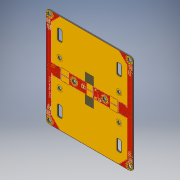
# Autodesk Inventor part: SolarPanel_PCB
Saved by Autodesk Inventor 2018 (Build 220112000, 112)
## iProperties
Created: 2018-11-29
Part Number: SolarPanel_PCB
Material: Epoxy Resin
Document SubType Name: Modeling
Designer: Bradley
Density: 1.14 g/cm^3
Appearance: Smooth - Dark Gray
Author: Bradley
Autodesk Inventor part; units mm, degrees
ref_plane "YZ Plane" through (0, 0, 0) normal (1, 0, 0) x (0, 1, 0)
ref_plane "XZ Plane" through (0, 0, 0) normal (0, 1, 0) x (-1, 0, 0)
ref_plane "XY Plane" through (0, 0, 0) normal (0, 0, 1) x (1, 0, 0)
sketch "Sketch1" plane through (0, 0, 0) normal (0, 1, 0) x (-1, 0, 0)
  line L0 (36.5, -45) -> (-36.5, -45)
  line L1 (-39.5, -42) -> (-39.5, 42)
  line L2 (-36.5, 45) -> (36.5, 45)
  line L3 (39.5, 42) -> (39.5, -42)
  line L4 (39.5, -45) -> (-39.5, 45) construction
  line L5 (-39.5, -45) -> (39.5, 45) construction
  arc A0 (39.5, 42) -> (36.5, 45) centre (36.5, 42) ccw
  arc A1 (36.5, -45) -> (39.5, -42) centre (36.5, -42) ccw
  arc A2 (-39.5, -42) -> (-36.5, -45) centre (-36.5, -42) ccw
  arc A3 (-36.5, 45) -> (-39.5, 42) centre (-36.5, 42) ccw
  circle A4 centre (36.5, 42) radius 1.65
  circle A5 centre (-36.5, 42) radius 1.65
  circle A6 centre (-36.5, -42) radius 1.65
  circle A7 centre (36.5, -42) radius 1.65
  line L6 (14, 0) -> (-14, 0) construction
  circle A8 centre (14, 0) radius 1.65
  circle A9 centre (-14, 0) radius 1.65
  line L7 (28, 35) -> (26, 35)
  line L8 (25, 34) -> (25, 26)
  line L9 (26, 25) -> (28, 25)
  line L10 (29, 26) -> (29, 34)
  line L11 (-26, 35) -> (-28, 35)
  line L12 (-29, 34) -> (-29, 26)
  line L13 (-28, 25) -> (-26, 25)
  line L14 (-25, 26) -> (-25, 34)
  line L15 (28, -25) -> (26, -25)
  line L16 (25, -26) -> (25, -34)
  line L17 (26, -35) -> (28, -35)
  line L18 (29, -34) -> (29, -26)
  line L19 (-26, -25) -> (-28, -25)
  line L20 (-29, -26) -> (-29, -34)
  line L21 (-28, -35) -> (-26, -35)
  line L22 (-25, -34) -> (-25, -26)
  line L23 (0, 45) -> (0, -45) construction
  arc A10 (29, 34) -> (28, 35) centre (28, 34) ccw
  arc A11 (26, 35) -> (25, 34) centre (26, 34) ccw
  arc A12 (25, 26) -> (26, 25) centre (26, 26) ccw
  arc A13 (28, 25) -> (29, 26) centre (28, 26) ccw
  arc A14 (26, -25) -> (25, -26) centre (26, -26) ccw
  arc A15 (29, -26) -> (28, -25) centre (28, -26) ccw
  arc A16 (28, -35) -> (29, -34) centre (28, -34) ccw
  arc A17 (25, -34) -> (26, -35) centre (26, -34) ccw
  arc A18 (-26, -35) -> (-25, -34) centre (-26, -34) ccw
  arc A19 (-26, 25) -> (-25, 26) centre (-26, 26) ccw
  arc A20 (-25, 34) -> (-26, 35) centre (-26, 34) ccw
  arc A21 (-28, 35) -> (-29, 34) centre (-28, 34) ccw
  arc A22 (-29, 26) -> (-28, 25) centre (-28, 26) ccw
  arc A23 (-28, -25) -> (-29, -26) centre (-28, -26) ccw
  arc A24 (-25, -26) -> (-26, -25) centre (-26, -26) ccw
  arc A25 (-29, -34) -> (-28, -35) centre (-28, -34) ccw
  point P0 (0, 0)
  point P1 (0, 0)
  point P2 (-25, 35)
  point P3 (-29, 25)
  point P4 (29, -25)
  point P5 (25, -35)
  point P6 (-25, -25)
  point P7 (-29, -35)
  dimension "d0" = 79
  dimension "d1" = 90
  dimension "d2" = 3
  dimension "d3" = 3.3
  dimension "d4" = 28
  dimension "d92" = 29
  dimension "d93" = 35
  dimension "d94" = 25
  dimension "d95" = 25
  dimension "d96" = 1
  constraints: 48 end point, 40 point on circle, 40 tangent, 28 point on line, 26 centre point, 23 equal radius, 10 parallel, 6 coincident, 6 horizontal, 6 midpoint, 5 perpendicular, 1 collinear, 3 other
  measures "d0" distance of L4.end L5.end
  measures "d1" distance of L5.end L4.start
  measures "d2" radius of A0
  measures "d3" diameter of A4
  measures "d4" distance of L6.start L6.end
  measures "d92" distance from line of L10 point (0, 0)
  measures "d93" distance from line of point (0, 0) L7
  measures "d94" distance from line of L9 point (0, 0)
  measures "d95" distance from line of point (0, 0) L8
  measures "d96" radius of A10
extrude "Extrusion1" add sketch "Sketch1" along normal mid plane 1
sketch "Sketch8" plane through (0, -0.5, 0) normal (0, -1, 0) x (1, 0, 0)
  line L0 (-39.5061, 45) -> (39.5061, 45) construction
  line L1 (39.5061, 45) -> (39.5061, -45) construction
  line L2 (39.5061, -45) -> (-39.5061, -45) construction
  line L3 (-39.5061, -45) -> (-39.5061, 45) construction
  line L4 (36.5, 45) -> (-36.5, 45) projected
  line L5 (-36.5, -45) -> (36.5, -45) projected
  point P0 (0, 0)
  point P1 (0, 45)
  constraints: 2 collinear, 2 midpoint, 2 other
decal "Decal3"
sketch "Sketch9" plane through (0, 0.5, 0) normal (0, 1, 0) x (1, 0, 0)
  line L0 (-36.5, -45) -> (36.5, -45) projected
  line L1 (36.5, 45) -> (-36.5, 45) projected
  line L2 (39.5061, -45) -> (-39.5061, -45) construction
  line L3 (-39.5061, -45) -> (-39.5061, 45) construction
  line L4 (-39.5061, 45) -> (39.5061, 45) construction
  line L5 (39.5061, 45) -> (39.5061, -45) construction
  point P0 (0, 0)
  point P1 (0, -45)
  point P2 (0, -45)
  constraints: 3 midpoint, 2 collinear, 2 other
decal "Decal4"
sketch "Sketch10" plane through (0, -0.5, 0) normal (0, -1, 0) x (1, 0, 0)
  point P0 (0, 0)
  point P1 (27, -12)
  point P2 (-27, -12)
  point P3 (-27, 12)
  point P4 (27, 12)
  constraints: 5 other
hole "Hole5" at (27, -0.5, -12) at (-27, -0.5, -12) at (-27, -0.5, 12) at (27, -0.5, 12) direction (0, 1, 0) diameter 3 end through all
sketch "Sketch11" plane through (0, -0.5, 0) normal (0, -1, 0) x (1, 0, 0)
  point P0 (0, 0)
  point P1 (-35.789, -39.813)
  point P2 (-37.211, -39.813)
  point P3 (-38.361, -40.648)
  point P4 (-38.8, -42)
  point P5 (-38.361, -43.352)
  point P6 (-37.211, -44.187)
  point P7 (-35.789, -44.187)
  point P8 (-34.639, -40.648)
  point P9 (-34.2, 42)
  point P10 (-34.639, 43.352)
  point P11 (-35.789, 44.187)
  point P12 (-37.211, 44.187)
  point P13 (-38.361, 43.352)
  point P14 (-38.8, 42)
  point P15 (-38.361, 40.648)
  point P16 (-37.211, 39.813)
  point P17 (-35.789, 39.813)
  point P18 (-34.639, 40.648)
  point P19 (38.8, 42)
  point P20 (38.361, 43.352)
  point P21 (37.211, 44.187)
  point P22 (35.789, 44.187)
  point P23 (34.639, 43.352)
  point P24 (34.2, 42)
  point P25 (34.639, 40.648)
  point P26 (35.789, 39.813)
  point P27 (37.211, 39.813)
  point P28 (38.361, 40.648)
  point P29 (-34.639, -43.352)
  point P30 (38.8, -42)
  point P31 (38.361, -40.648)
  point P32 (37.211, -39.813)
  point P33 (35.789, -39.813)
  point P34 (34.639, -40.648)
  point P35 (34.2, -42)
  point P36 (34.639, -43.352)
  point P37 (35.789, -44.187)
  point P38 (37.211, -44.187)
  point P39 (38.361, -43.352)
  point P40 (-34.2, -42)
  point P41 (-11.7, 0)
  point P42 (-12.139, 1.352)
  point P43 (-14.711, 2.187)
  point P44 (-15.861, 1.352)
  point P45 (-16.3, 0)
  point P46 (-15.861, -1.352)
  point P47 (-14.711, -2.187)
  point P48 (-13.289, -2.187)
  point P49 (-12.139, -1.352)
  point P50 (-13.289, 2.187)
  point P51 (16.3, 0)
  point P52 (15.861, 1.352)
  point P53 (14.711, 2.187)
  point P54 (13.289, 2.187)
  point P55 (12.139, 1.352)
  point P56 (11.7, 0)
  point P57 (12.139, -1.352)
  point P58 (13.289, -2.187)
  point P59 (14.711, -2.187)
  point P60 (15.861, -1.352)
  constraints: 61 other
hole "Hole6" at (-35.789, -0.5, -39.813) at (-37.211, -0.5, -39.813) at (-38.361, -0.5, -40.648) at (-38.8, -0.5, -42) at (-38.361, -0.5, -43.352) at (-37.211, -0.5, -44.187) at (-35.789, -0.5, -44.187) at (-34.639, -0.5, -40.648) at (-34.2, -0.5, 42) at (-34.639, -0.5, 43.352) at (-35.789, -0.5, 44.187) at (-37.211, -0.5, 44.187) at (-38.361, -0.5, 43.352) at (-38.8, -0.5, 42) at (-38.361, -0.5, 40.648) at (-37.211, -0.5, 39.813) at (-35.789, -0.5, 39.813) at (-34.639, -0.5, 40.648) at (38.8, -0.5, 42) at (38.361, -0.5, 43.352) at (37.211, -0.5, 44.187) at (35.789, -0.5, 44.187) at (34.639, -0.5, 43.352) at (34.2, -0.5, 42) at (34.639, -0.5, 40.648) at (35.789, -0.5, 39.813) at (37.211, -0.5, 39.813) at (38.361, -0.5, 40.648) at (-34.639, -0.5, -43.352) at (38.8, -0.5, -42) at (38.361, -0.5, -40.648) at (37.211, -0.5, -39.813) at (35.789, -0.5, -39.813) at (34.639, -0.5, -40.648) at (34.2, -0.5, -42) at (34.639, -0.5, -43.352) at (35.789, -0.5, -44.187) at (37.211, -0.5, -44.187) at (38.361, -0.5, -43.352) at (-34.2, -0.5, -42) at (-11.7, -0.5, 0) at (-12.139, -0.5, 1.352) at (-14.711, -0.5, 2.187) at (-15.861, -0.5, 1.352) at (-16.3, -0.5, 0) at (-15.861, -0.5, -1.352) at (-14.711, -0.5, -2.187) at (-13.289, -0.5, -2.187) at (-12.139, -0.5, -1.352) at (-13.289, -0.5, 2.187) direction (0, 1, 0) diameter 0.45 end through all and at (16.3, -0.5, 0) (15.861, -0.5, 1.352) (14.711, -0.5, 2.187) (13.289, -0.5, 2.187) (12.139, -0.5, 1.352) (11.7, -0.5, 0) (12.139, -0.5, -1.352) (13.289, -0.5, -2.187) (14.711, -0.5, -2.187) (15.861, -0.5, -1.352)
sketch "Sketch12" plane through (0, -0.5, 0) normal (0, -1, 0) x (1, 0, 0)
  point P0 (0, 0)
  point P1 (38.14, 1.295)
  point P2 (35.25, 34)
  point P3 (-36.49, 34.246)
  point P4 (-37.82, 2.5)
  point P5 (-9.75, 4.25)
  point P6 (-28.824, -2.335)
  point P7 (-7.75, -0.06)
  point P8 (-36, -33.75)
  point P9 (29.21, -4)
  point P10 (29.21, -2.92)
  point P11 (22.25, 4.75)
  point P12 (-2, 4.75)
  point P13 (5, 4.25)
  point P14 (-22.25, -4.75)
  point P15 (2, -4.75)
  point P16 (18.25, -4)
  point P17 (-18.25, 4)
  point P18 (-38.435, 0.565)
  point P19 (-38.435, -0.565)
  point P20 (38.46, -0.54)
  point P21 (38.46, 0.54)
  point P22 (-4.75, -3.5)
  point P23 (-37.82, -2.5)
  point P24 (34.25, -37.84)
  point P25 (-29.54, -4.25)
  point P26 (-29.555, 4.25)
  point P27 (-28.78, -4.25)
  point P28 (-18.25, 2.75)
  point P29 (5.5, 0)
  point P30 (33, -0.75)
  point P31 (28.5, -0.75)
  point P32 (-26.49, 4.25)
  point P33 (-26.21, 2.68)
  point P34 (10.24, -4.5)
  point P35 (29.2, 3.68)
  point P36 (30.28, 4.75)
  point P37 (4, 3.49)
  point P38 (36.74, -34.496)
  point P39 (37.82, -2.55)
  point P40 (37.82, 2.5)
  point P41 (36.5, 32.25)
  point P42 (-37.25, 34.25)
  point P43 (-38.14, 1.35)
  point P44 (-38.14, -1.35)
  point P45 (-29, -1.5)
  point P46 (-7.75, 0.75)
  point P47 (-36, -34.51)
  point P48 (-35, -26.25)
  point P49 (7.75, 3.49)
  point P50 (10.75, -1.5)
  point P51 (-30.575, -0.675)
  point P52 (-29.75, -2)
  point P53 (-8.75, -2.74)
  point P54 (-8.75, 3.145)
  point P55 (-28.77, 4.25)
  point P56 (-28.02, -4.25)
  point P57 (23.25, 0)
  point P58 (-28.486, -0.865)
  point P59 (33.375, -2.375)
  point P60 (27.96, -4)
  point P61 (26.24, -4.246)
  point P62 (34.007, -2.993)
  point P63 (27, -4.25)
  point P64 (18.246, -3.24)
  point P65 (30.28, -4.457)
  point P66 (-27.25, 4.254)
  point P67 (-26.5, -4.254)
  point P68 (-28.01, 4.25)
  point P69 (-27.26, -4.25)
  point P70 (-29.544, 3.44)
  point P71 (-28.014, -2.335)
  point P72 (-7.75, -0.87)
  point P73 (-35.75, -29.75)
  point P74 (-35.73, 34.243)
  point P75 (35.75, 30)
  point P76 (35.98, -34.493)
  point P77 (37.5, -34.5)
  point P78 (38.14, -1.295)
  constraints: 79 other
hole "Hole7" at (38.14, -0.5, 1.295) at (35.25, -0.5, 34) at (-36.49, -0.5, 34.246) at (-37.82, -0.5, 2.5) at (-9.75, -0.5, 4.25) at (-28.824, -0.5, -2.335) at (-7.75, -0.5, -0.06) at (-36, -0.5, -33.75) at (29.21, -0.5, -4) at (29.21, -0.5, -2.92) at (22.25, -0.5, 4.75) at (-2, -0.5, 4.75) at (5, -0.5, 4.25) at (-22.25, -0.5, -4.75) at (2, -0.5, -4.75) at (18.25, -0.5, -4) at (-18.25, -0.5, 4) at (-38.435, -0.5, 0.565) at (-38.435, -0.5, -0.565) at (38.46, -0.5, -0.54) at (38.46, -0.5, 0.54) at (-4.75, -0.5, -3.5) at (-37.82, -0.5, -2.5) at (34.25, -0.5, -37.84) at (-29.54, -0.5, -4.25) at (-29.555, -0.5, 4.25) at (-28.78, -0.5, -4.25) at (-18.25, -0.5, 2.75) at (5.5, -0.5, 0) at (33, -0.5, -0.75) at (28.5, -0.5, -0.75) at (-26.49, -0.5, 4.25) at (-26.21, -0.5, 2.68) at (10.24, -0.5, -4.5) at (29.2, -0.5, 3.68) at (30.28, -0.5, 4.75) at (4, -0.5, 3.49) at (36.74, -0.5, -34.496) at (37.82, -0.5, -2.55) at (37.82, -0.5, 2.5) at (36.5, -0.5, 32.25) at (-37.25, -0.5, 34.25) at (-38.14, -0.5, 1.35) at (-38.14, -0.5, -1.35) at (-29, -0.5, -1.5) at (-7.75, -0.5, 0.75) at (-36, -0.5, -34.51) at (-35, -0.5, -26.25) at (7.75, -0.5, 3.49) at (10.75, -0.5, -1.5) direction (0, 1, 0) diameter 0.3 end through all and at (-30.575, -0.5, -0.675) (-29.75, -0.5, -2) (-8.75, -0.5, -2.74) (-8.75, -0.5, 3.145) (-28.77, -0.5, 4.25) (-28.02, -0.5, -4.25) (23.25, -0.5, 0) (-28.486, -0.5, -0.865) (33.375, -0.5, -2.375) (27.96, -0.5, -4) (26.24, -0.5, -4.246) (34.007, -0.5, -2.993) (27, -0.5, -4.25) (18.246, -0.5, -3.24) (30.28, -0.5, -4.457) (-27.25, -0.5, 4.254) (-26.5, -0.5, -4.254) (-28.01, -0.5, 4.25) (-27.26, -0.5, -4.25) (-29.544, -0.5, 3.44) (-28.014, -0.5, -2.335) (-7.75, -0.5, -0.87) (-35.75, -0.5, -29.75) (-35.73, -0.5, 34.243) (35.75, -0.5, 30) (35.98, -0.5, -34.493) (37.5, -0.5, -34.5) (38.14, -0.5, -1.295)
body "Solid1"
